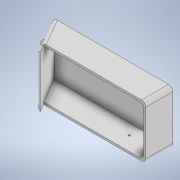
# Autodesk Inventor part: Case
Saved by Autodesk Inventor 2021 (Build 250183000, 183)
## iProperties
Created: 2020-08-28
Part Number: Case
Material: Generisch
Document SubType Name: Modeling
Designer: michox
Density: 1 g/cm^3
Appearance: Vorgabe
Author: michox
Autodesk Inventor part; units mm, degrees
ref_plane "YZ Plane" through (0, 0, 0) normal (1, 0, 0) x (0, 1, 0)
ref_plane "XZ Plane" through (0, 0, 0) normal (0, 1, 0) x (-1, 0, 0)
ref_plane "XY Plane" through (0, 0, 0) normal (0, 0, 1) x (1, 0, 0)
sketch "Skizze1" plane through (0, 0, 0) normal (0, 0, 1) x (1, 0, 0)
  line L0 (0, 0) -> (135, 0)
  line L1 (135, 0) -> (135, -60)
  line L2 (135, -60) -> (0, -60)
  line L3 (0, -60) -> (0, 0)
  dimension "d0" = 135
  dimension "d1" = 60
  constraints: 8 end point, 2 parallel, 1 horizontal, 1 perpendicular
  measures "d0" distance of L1.end L2.end
  measures "d1" distance of L0.end L1.end
extrude "Extrusion1" add sketch "Skizze1" along normal blind 40
chamfer "Fase1" distance 38 angle 30 1 edges at (0, -30, 40) measured on face at (0, -20, 13.3333)
shell "Wandung1" thickness 2.5 removed faces 1 at (59.626207, -20, 40)
sketch "Skizze2" plane through (0, 0, 40) normal (0, 0, 1) x (1, 0, 0)
  line L0 (24.826062, -57.5) -> (24.826062, -2.5)
  line L1 (24.826062, -2.5) -> (24.826062, 0)
  line L2 (24.826062, 0) -> (24.826062, -57.5)
  line L3 (24.826062, -57.5) -> (24.826062, -60)
  line L4 (32.285534, -57.5) -> (32.285534, -2.5)
  line L5 (32.285534, -2.5) -> (132.5, -2.5)
  line L6 (132.5, -2.5) -> (132.5, -57.5)
  line L7 (132.5, -57.5) -> (32.285534, -57.5)
  line L8 (21.290528, -60) -> (21.290528, 0)
  line L9 (21.290528, -60) -> (24.826062, -60)
  line L10 (135.042932, -60) -> (135.042932, 0)
  line L11 (135.042932, 0) -> (24.826062, 0)
  line L12 (24.826062, -60) -> (135.042932, -60)
  line L13 (24.826062, 0) -> (21.290528, 0)
  point P0 (0, 0)
  point P1 (32.285534, -2.5)
  constraints: 26 end point, 1 collinear, 1 point on line, 1 vertical
extrude "Extrusion2" cut sketch "Skizze2" against normal blind 9.5 contours L0 L1 L11 L10 L12 L3
sketch "Skizze3" plane through (0, -60, 0) normal (0, -1, 0) x (1, 0, 0)
  point P0 (0, 0)
  point P1 (100.666226, 14.858037)
hole "Bohrung1" at (100.666226, -60, 14.858037) direction (0, 1, 0) diameter 2 depth 8 tip angle 118
sketch "Skizze4" plane through (132.5, -57.5, 2.5) normal (-1, 0, 0) x (0, 0, 1)
  line L0 (22.221117, 33.89428) -> (25.5, 33.89428)
  line L1 (25.5, 33.89428) -> (25.5, 21.10572)
  line L2 (25.5, 21.10572) -> (22.221117, 21.10572)
  line L3 (22.221117, 21.10572) -> (22.221117, 33.89428)
  line L4 (0, 0) -> (0, 55)
  line L5 (0, 27.5) -> (28, 27.5)
  line L6 (28, 0) -> (28, 55)
  line L7 (28, 57.5) -> (28, -2.5)
  point P0 (-2.5, 57.5)
  dimension "d22" = 2.5
  constraints: 10 end point, 2 midpoint, 2 parallel, 1 horizontal, 1 perpendicular, 1 other
  measures "d22" distance between parallel lines of L1 L7
extrude "Extrusion3" cut sketch "Skizze4" against normal blind 1
sketch "Skizze5" plane through (0, -60, 0) normal (0, -1, 0) x (1, 0, 0)
  line L0 (132.5, 30.5) -> (24.826062, 30.5)
  line L1 (32.285534, 30.5) -> (19.341234, 30.5)
  line L2 (19.341234, 30.5) -> (24.826062, 40)
  line L3 (3.175426, 2.5) -> (24.826062, 40)
  line L4 (24.826062, 40) -> (32.013518, 40)
  line L5 (32.013518, 40) -> (32.013518, 30.5)
  point P0 (0, 0)
  point P1 (2.5, 4.827159)
  point P2 (23.251035, 30.965501)
  point P3 (127.540528, 30.5)
  point P4 (24.826062, 40)
  constraints: 8 end point, 2 horizontal, 1 parallel, 1 perpendicular, 6 other
extrude "Extrusion4" cut sketch "Skizze5" against normal through all
sketch "Skizze6" plane through (0, -60, 0) normal (0, -1, 0) x (1, 0, 0)
  circle A0 centre (100.666226, 14.858037) radius 1
  line L0 (124.166226, 9.858037) -> (123.166226, 9.858037)
  line L1 (123.166226, 9.858037) -> (123.166226, 19.858037)
  line L2 (123.166226, 19.858037) -> (124.166226, 19.858037)
  line L3 (124.166226, 19.858037) -> (124.166226, 9.858037)
  line L4 (100.666226, 14.858037) -> (116.026843, 14.858037)
  point P0 (0, 0)
  dimension "d23" = 1
  dimension "d24" = 10
  dimension "d25" = 22.5
  constraints: 10 end point, 2 horizontal, 2 parallel, 1 perpendicular, 1 other
  measures "d23" distance of L1.end L2.end
  measures "d24" distance of L0.end L1.end
  measures "d25" distance from line of L4.start L1
extrude "Extrusion5" cut sketch "Skizze6" against normal up to surface (2.5 mm away) contours L0 L1 L2 L3
sketch "Skizze7" plane through (0, 0, 0) normal (0, 0, -1) x (-1, 0, 0)
  line L0 (0, -36) -> (6.514704, -36)
  line L1 (12.514704, -30) -> (12.514704, -30)
  line L2 (6.514704, -24) -> (0, -24)
  line L3 (0, -24) -> (0, -36)
  line L4 (-21.93931, -60) -> (-21.93931, 0)
  line L5 (-21.93931, -30) -> (18.562445, -30)
  circle A0 centre (6.514704, -30) radius 3
  arc A1 (6.514704, -36) -> (12.514704, -30) centre (6.514704, -30) ccw
  arc A2 (12.514704, -30) -> (6.514704, -24) centre (6.514704, -30) ccw
  point P0 (0, 0)
  point P1 (12.514704, -30)
  dimension "d28" = 6
  dimension "d29" = 6
  dimension "d30" = 6
  dimension "d31" = 6
  constraints: 10 end point, 4 point on circle, 4 tangent, 3 centre point, 2 horizontal, 2 parallel, 1 concentric, 1 midpoint, 1 perpendicular, 1 point on line, 1 other
  measures "d28" diameter of A0
  measures "d29" radius of A1
  measures "d30" distance from line of L0 A0.centre
  measures "d31" distance from line of L1 A0.centre
extrude "Extrusion6" add sketch "Skizze7" against normal blind 2 contours L3 L5 A0 A1 L0 | L3 L2 A2 L5 A0
fillet "Rundung1" radius 4.75 2 edges at (0, -24, 1) (0, -36, 1)
fillet "Rundung2" radius 4.75 7 edges at (21.9393, -30, 40) (10.9697, -60, 21) (10.9697, 0, 21) (135, 0, 15.25) (135, -60, 15.25) (132.5, -57.5, 16.5) (132.5, -2.5, 16.5)
